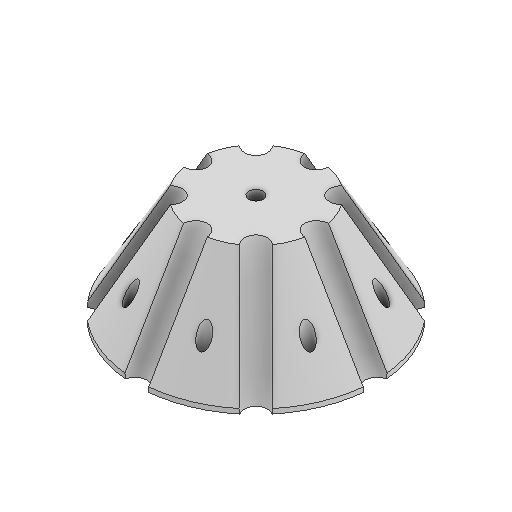
# Autodesk Inventor part: 3DP_ASA_Bottom_Cone_Bottom_Half
Saved by Autodesk Inventor 2026.1 (Build 301233000, 233)
## iProperties
Created: 2025-06-19
Part Number: 3DP_ASA_Bottom_Cone_Bottom_Half
Material: Generic
Document SubType Name: Modeling
Designer: User
Density: 1 g/cm^3
Appearance: Default
Author: User
Autodesk Inventor part; units mm, degrees
ref_plane "YZ Plane" through (0, 0, 0) normal (1, 0, 0) x (0, 1, 0)
ref_plane "XZ Plane" through (0, 0, 0) normal (0, 1, 0) x (-1, 0, 0)
sketch "Sketch1" plane through (0, 0, 0) normal (0, 0, 1) x (1, 0, 0)
  line L0 (0, 53.9615) -> (-20, 53.9615)
  line L1 (-20, 53.9615) -> (-50, 2)
  line L2 (-50, 2) -> (-50, 0)
  line L3 (-50, 0) -> (0, 0)
  line L4 (0, 0) -> (0, 53.9615)
  line L5 (0, -10.7923) -> (0, 64.7538) projected
  dimension "d0" = 50
  dimension "d2" = 20
  dimension "d3" = 30
  dimension "d4" = 2
  dimension "d5" = 53.9615
  constraints: 10 end point, 2 perpendicular, 1 horizontal, 1 vertical
  measures "d0" distance between parallel lines of L4 L2
  measures "d2" distance of L0.start L0.end
  measures "d3" angle of L4 L1
  measures "d4" distance of L1.end L2.end
  measures "d5" distance between parallel lines of L3 L0
revolve "Revolution1" add sketch "Sketch1" angle 360 about axis through (0, -10, 0) along (0, 1, 0)
sketch "Sketch2" plane through (0, 53.9615, 0) normal (0, 1, 0) x (1, 0, 0)
  circle A0 centre (0, 0) radius 20 projected
  line L0 (-20, 26.6864) -> (-20, -29.355)
  dimension "d7" = 40
  dimension "d8" = 20
  constraints: 2 end point, 1 vertical
  measures "d7" diameter of A0
  measures "d8" distance from line of point (0, 0) L0
ref_plane "Work Plane1" through (-20, 53.9615, -26.6864) normal (-0.5, -0.866, 0) x (0, 0, 1)
sketch "Sketch3" plane through (-20, 53.9615, -26.6864) normal (-0.5, -0.866, 0) x (0, 0, 1)
  ellipse E0 centre (26.6864, -43.3013) end of major axis (-23.3136, -43.3013) minor radius 43.3013 projected
  circle A0 centre (26.6864, 0.25) radius 5
  point P0 (26.6864, -44.3013)
  point P1 (26.6864, 0)
  dimension "d11" = 0.25
  dimension "d12" = 10
  constraints: 1 centre point, 1 coincident, 1 vertical alignment, 1 other
  measures "d11" distance of point (26.686, 0) point (26.686, 0.25)
  measures "d12" diameter of A0
extrude "Extrusion1" cut sketch "Sketch3" along normal mid plane 200 contours A0 E0 | E0 A0 picked at (25.0675, -1.4032) picked at (28.4242, 1.4636)
pattern_circular "Circular Pattern1" count 8 over 360 about axis through (0, -10, 0) along (0, 1, 0) of "Extrusion1"
sketch "Sketch4" plane through (0, 53.9615, 0) normal (0, 1, 0) x (0.9239, 0, 0.3827)
  point P0 (0, 0)
  point P1 (0, 0)
  constraints: 1 coincident
hole "Hole1" at (0, 53.9615, 0) direction (0, -1, 0) diameter 6 end through all
sketch "Sketch5" plane through (0, 0, 0) normal (0, -1, 0) x (0.9239, 0, -0.3827)
  circle A0 centre (0, 0) radius 3 projected
  point P0 (0, 40)
  dimension "d26" = 40
  measures "d26" distance of point (0, 0) point (0, 40)
hole "Hole2" at (15.3073, 0, 36.9552) direction (0, 1, 0) diameter 5 end through all
pattern_circular "Circular Pattern2" count 8 over 360 about axis through (0, -10, 0) along (0, 1, 0) of "Hole2"
sketch "Sketch6" plane through (0, 53.9615, 0) normal (0, 1, 0) x (0.9239, 0, 0.3827)
  circle A0 centre (0, 0) radius 3 projected
  circle A1 centre (0, 0) radius 50
  dimension "d37" = 100
  constraints: 1 centre point, 1 coincident
  measures "d37" diameter of A1
extrude "Extrusion2" cut sketch "Sketch6" against normal blind 10
sketch "Sketch7" plane through (0, 0, 0) normal (0, -1, 0) x (0.9239, 0, -0.3827)
  circle A0 centre (0, 0) radius 3 projected
  circle A1 centre (0, 0) radius 15.1
  dimension "d40" = 30.2
  constraints: 1 centre point, 1 coincident
  measures "d40" diameter of A1
extrude "Extrusion3" cut sketch "Sketch7" against normal blind 20
equation "\"d8\" = 0.5 * d7"
body "Solid1"
